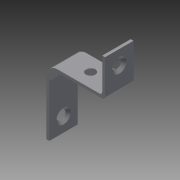
# Autodesk Inventor part: bracket
Saved by Autodesk Inventor 2014 (Build 180170000, 170)
## iProperties
Created: 2013-10-13
Part Number: bracket
Material: Generic
Document SubType Name: Modeling
Designer: david
Density: 1 g/cm^3
Appearance: Default
Author: david
Autodesk Inventor part; units mm, degrees
ref_plane "YZ Plane" through (0, 0, 0) normal (1, 0, 0) x (0, 1, 0)
ref_plane "XZ Plane" through (0, 0, 0) normal (0, 1, 0) x (-1, 0, 0)
ref_plane "XY Plane" through (0, 0, 0) normal (0, 0, 1) x (1, 0, 0)
sketch "Sketch1" plane through (0, 0, 0) normal (0, 0, 1) x (1, 0, 0)
  line L0 (1.5875, 14.0208) -> (1.5875, 42.8625)
  line L1 (0, 44.45) -> (0, 14.0208)
  line L2 (6.35, 50.8) -> (31.0388, 50.8)
  line L3 (32.6263, 49.2125) -> (7.9375, 49.2125)
  arc A0 (6.35, 50.8) -> (0, 44.45) centre (6.35, 44.45) ccw
  line L4 (1.5875, 42.8625) -> (7.9375, 49.2125)
  line L5 (31.0388, 50.8) -> (31.0388, 69.85)
  line L6 (32.6263, 50.8) -> (32.6263, 69.85)
  line L7 (31.0388, 69.85) -> (32.6263, 69.85)
  line L8 (32.6263, 50.8) -> (32.6263, 49.2125)
  line L9 (0, 14.0208) -> (1.5875, 14.0208)
  point P0 (0, 0)
  point P1 (1.8599, 48.9401)
  point P2 (4.7625, 46.0375)
  dimension "d7" = 1.5875
  dimension "d8" = 19.05
  dimension "d48" = 24.6888
  constraints: 20 end point, 4 parallel, 4 perpendicular, 3 point on circle, 2 horizontal, 1 centre point, 1 midpoint, 1 tangent, 3 other
  measures "d7" distance between parallel lines of L6 L5
  measures "d8" distance of L2.end L5.end
  measures "d48" distance of L2.start L2.end
extrude "Extrusion1" add sketch "Sketch1" along normal blind 15.875
fillet "Fillet1" radius 1.5875 2 edges at (31.0388, 50.8, 7.9375) (32.6263, 49.2125, 7.9375)
sketch "Sketch2" plane through (32.6263, 69.85, 15.875) normal (1, 0, 0) x (0, 0, -1)
  line L0 (15.875, 0) -> (0, 0) projected
  point P0 (15.875, -69.85)
  point P1 (7.9375, -7.9375)
  dimension "d12" = 7.9375
  measures "d12" distance from line of L0 point (7.938, -7.938)
sketch "Sketch5" plane through (7.9375, 49.2125, 0) normal (0, -1, 0) x (1, 0, 0)
  point P0 (-7.9375, 0)
  point P1 (8.7312, 7.9375)
sketch "Sketch6" plane through (1.5875, 14.0208, 0) normal (1, 0, 0) x (0, 0, -1)
  line L0 (0, 0) -> (-15.875, 0) projected
  line L1 (0, 0) -> (0, 28.8417) projected
  line L2 (0, 28.8417) -> (-15.875, 28.8417) projected
  line L3 (-15.875, 0) -> (-15.875, 28.8417) projected
  line L4 (0, 0) -> (-15.875, 0) projected
  point P0 (-7.9375, 7.9375)
  point P1 (-7.9375, 30.1625)
  dimension "d15" = 7.9375
  measures "d15" distance from line of L0 point (-7.938, 7.938)
hole "Hole2" at (16.6687, 49.2125, 7.9375) direction (0, 1, 0) diameter 4.7625 end through all countersink diameter 7.9375 countersink angle 82
hole "Hole3" at (32.6263, 61.9125, 7.9375) direction (-1, 0, 0) diameter 4.7625 end through all countersink diameter 7.9375 countersink angle 82
hole "Hole4" at (1.5875, 21.9583, 7.9375) direction (-1, 0, 0) diameter 4.7625 end through all countersink diameter 7.9375 countersink angle 82
body "Solid1"
